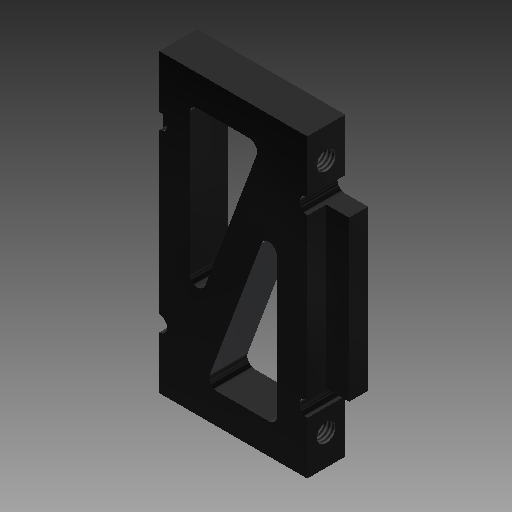
# Autodesk Inventor part: 胴体_メインフレーム_1_12
Saved by Autodesk Inventor 2018 (Build 220112000, 112)
## iProperties
Created: 2016-05-21
Part Number: 胴体_メインフレーム_1_12
Material: アセタール樹脂、黒
Document SubType Name: Modeling
Designer: hiroaki
Density: 1.425 g/cm^3
Appearance: 滑らか - 黒
Mass: 4.06026 g
Surface Area: 24.9325 cm^2
Volume: 2.84931 cm^3
Author: hiroaki
Autodesk Inventor part; units mm, degrees
ref_plane "YZ Plane" through (0, 0, 0) normal (1, 0, 0) x (0, 1, 0)
ref_plane "XZ Plane" through (0, 0, 0) normal (0, 1, 0) x (-1, 0, 0)
ref_plane "XY Plane" through (0, 0, 0) normal (0, 0, 1) x (1, 0, 0)
sketch "スケッチ1" plane through (0, 0, 0) normal (0, 0, 1) x (1, 0, 0)
  line L0 (-9.75, -19.5) -> (9.75, -19.5) construction
  line L1 (9.75, -19.5) -> (9.75, 19.5) construction
  line L2 (9.75, 19.5) -> (-9.75, 19.5) construction
  line L3 (-9.75, 19.5) -> (-9.75, -19.5) construction
  line L4 (-9.75, -19.5) -> (9.75, 19.5) construction
  line L5 (9.75, -19.5) -> (-9.75, 19.5) construction
  line L6 (-9.75, 10.5) -> (-9.75, 19.5) construction
  line L7 (-9.75, 19.5) -> (9.75, 19.5)
  line L8 (9.75, 19.5) -> (9.75, 10.5) construction
  line L9 (-9.75, 10.5) -> (-11.75, 10.5)
  line L10 (-11.75, 10.5) -> (-11.75, -10.5)
  line L11 (-11.75, -10.5) -> (-9.75, -10.5)
  line L12 (-9.75, -10.5) -> (-9.75, -19.5) construction
  line L13 (-9.75, -19.5) -> (9.75, -19.5)
  line L14 (9.75, -19.5) -> (9.75, -10.5) construction
  line L15 (9.75, -10.5) -> (12.75, -10.5)
  line L16 (12.75, -10.5) -> (12.75, 10.5)
  line L17 (12.75, 10.5) -> (9.75, 10.5)
  line L18 (0, 0) -> (12.75, 0) construction
  circle A0 centre (-9.75, 11.55) radius 1.05 construction
  circle A1 centre (-9.75, -11.55) radius 1.05 construction
  circle A2 centre (9.75, 11.55) radius 1.05 construction
  circle A3 centre (9.75, -11.55) radius 1.05 construction
  line L19 (-9.75, 19.5) -> (-9.75, 12.6)
  arc A4 (-9.75, 10.5) -> (-9.75, 12.6) centre (-9.75, 11.55) ccw
  arc A5 (-9.75, -12.6) -> (-9.75, -10.5) centre (-9.75, -11.55) ccw
  line L20 (-9.75, -12.6) -> (-9.75, -19.5)
  line L21 (9.75, 12.6) -> (9.75, 19.5)
  arc A6 (9.75, 12.6) -> (9.75, 10.5) centre (9.75, 11.55) ccw
  line L22 (9.75, -12.6) -> (9.75, -19.5)
  arc A7 (9.75, -10.5) -> (9.75, -12.6) centre (9.75, -11.55) ccw
  dimension "d21" = 2
  dimension "d23" = 3
  dimension "d30" = 19.5
  dimension "d48" = 9
  dimension "d49" = 39
  dimension "d50" = 2.1
  constraints: 46 end point, 16 point on circle, 9 perpendicular, 8 centre point, 8 collinear, 8 point on line, 6 equal radius, 5 parallel, 3 midpoint, 2 horizontal alignment, 2 tangent, 2 vertical, 1 coincident, 1 horizontal
  measures "d21" distance between parallel lines of L10 L3
  measures "d23" distance between parallel lines of L16 L1
  measures "d30" distance between parallel lines of L1 L3
  measures "d48" distance between parallel lines of L2 L9
  measures "d49" distance of L2.end L0.start
  measures "d50" diameter of A0
extrude "押し出し1" add sketch "スケッチ1" along normal blind 5
sketch "スケッチ2" plane through (9.75, -19.5, 0) normal (1, 0, 0) x (0, 0, -1)
  line L0 (0, 0) -> (-5, 0) projected
  line L1 (0, 39) -> (-5, 39) projected
  point P0 (0, 19.5)
  point P1 (-2.5, 4)
  point P2 (-2.5, 35)
  point P3 (-2.5, 0)
  dimension "d53" = 4
  dimension "d54" = 4
  constraints: 2 vertical alignment, 1 midpoint
  measures "d53" distance from line of L0 point (-2.5, 4)
  measures "d54" distance from line of L1 point (-2.5, 35)
hole "穴1" at (9.75, -15.5, 2.5) at (9.75, 15.5, 2.5) direction (-1, 0, 0) diameter 2.459 depth 2.5 tip angle 118 thread size "M3x0.5" class "6H" standard "ISO Metric profile"
mirror "ミラー1" about plane through (0, 0, 0) normal (1, 0, 0) of "穴1"
sketch "スケッチ3" plane through (0, 0, 5) normal (0, 0, 1) x (1, 0, 0)
  line L0 (9.75, 12.6) -> (9.75, 19.5) projected
  line L1 (-9.75, 19.5) -> (-9.75, 12.6) projected
  line L2 (-14.3307, 15.6684) -> (-9.75, 15.6684)
  line L3 (-9.75, 15.6684) -> (-9.75, -16.7148)
  line L4 (-9.75, -16.7148) -> (-14.3307, -16.7148)
  line L5 (-14.3307, -16.7148) -> (-14.3307, 15.6684)
  line L6 (15.2214, 11.55) -> (9.75, 11.55)
  line L7 (9.75, 11.55) -> (9.75, -15.9078)
  line L8 (9.75, -15.9078) -> (15.2214, -15.9078)
  line L9 (15.2214, -15.9078) -> (15.2214, 11.55)
  point P0 (0, 0)
  constraints: 16 end point, 4 parallel, 2 collinear, 2 horizontal, 2 perpendicular
extrude "押し出し2" cut sketch "スケッチ3" against normal blind 2.5
sketch "スケッチ4" plane through (0, 0, 5) normal (0, 0, 1) x (1, 0, 0)
  line L0 (9.75, 12.6) -> (9.75, 19.5) projected
  line L1 (9.75, 19.5) -> (-9.75, 19.5) projected
  line L2 (-9.75, -12.6) -> (-9.75, -19.5) projected
  line L3 (-9.75, -19.5) -> (9.75, -19.5) projected
  line L4 (-5.75, 15.5) -> (5.75, 15.5) construction
  line L5 (5.75, 15.5) -> (5.75, -15.5) construction
  line L6 (5.75, -15.5) -> (-5.75, -15.5) construction
  line L7 (-5.75, -15.5) -> (-5.75, 15.5) construction
  line L8 (5.75, 15.5) -> (-5.75, -15.5) construction
  line L9 (3.6168, 15.5) -> (-5.75, 15.5)
  line L10 (-5.75, 15.5) -> (-5.75, -9.7497)
  line L11 (-5.75, -9.7497) -> (3.6168, 15.5)
  line L12 (-3.6168, -15.5) -> (5.75, -15.5)
  line L13 (5.75, -15.5) -> (5.75, 9.7497)
  line L14 (5.75, 9.7497) -> (-3.6168, -15.5)
  point P0 (0, 0)
  dimension "d64" = 4
  dimension "d65" = 4
  dimension "d66" = 4
  dimension "d67" = 4
  dimension "d68" = 4
  constraints: 22 end point, 4 collinear, 4 parallel, 2 horizontal, 2 perpendicular, 1 vertical, 1 other
  measures "d64" distance between parallel lines of L14 L11
  measures "d65" distance between parallel lines of L1 L4
  measures "d66" distance between parallel lines of L3 L6
  measures "d67" distance between parallel lines of L2 L7
  measures "d68" distance between parallel lines of L0 L5
extrude "押し出し3" cut sketch "スケッチ4" against normal blind 5
fillet "フィレット1" radius 1.05 6 edges at (-3.6168, -15.5, 2.5) (-5.75, 15.5, 2.5) (3.6168, 15.5, 2.5) (5.75, 9.7497, 2.5) (-5.75, -9.7497, 2.5) (5.75, -15.5, 2.5)
equation "\"d48\" = d26 + d35"
equation "\"d49\" = d38"
equation "\"d53\" = d35"
equation "\"d54\" = d53"
equation "\"d66\" = d65"
equation "\"d68\" = d67"
equation "\"d26\" = 5"
equation "\"d35\" = 4"
equation "\"d38\" = 39"
